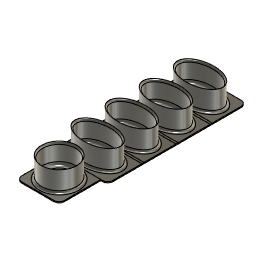
gluboost-organizer (Autodesk Fusion 360 design; units mm, degrees)
Autodesk Fusion 360 part; units mm, degrees
sketch "Sketch1" plane through (0, 0, 0) normal (0, 0, 1) x (1, 0, 0)
  ellipse E0 centre (0, 0) end of major axis (25.4, 0) minor radius 14.986
  line L0 (-25.4, 0) -> (25.4, 0)
  line L1 (0, -14.986) -> (0, 14.986)
  line L2 (33.6277, 21.621) -> (-33.6277, 21.621)
  line L3 (-33.6277, 21.621) -> (-33.6277, -21.621)
  line L4 (-33.6277, -21.621) -> (33.6277, -21.621)
  line L5 (33.6277, -21.621) -> (33.6277, 21.621)
  line L6 (33.6277, 21.621) -> (-33.6277, -21.621) construction
  line L7 (-33.6277, 21.621) -> (33.6277, -21.621) construction
  ellipse E1 centre (0, 0) end of major axis (27.1057, 0) minor radius 16.4243
  line L8 (-27.1057, 0) -> (27.1057, 0)
  line L9 (0, -16.4243) -> (0, 16.4243)
  line L10 (-25.4, -20.3918) -> (25.4, -71.1918) construction
  line L11 (25.4, -20.3918) -> (-25.4, -20.3918)
  circle A0 centre (0, -45.7918) radius 19.685
  line L12 (25.4, -71.1918) -> (25.4, -20.3918)
  line L13 (25.4, -20.3918) -> (-25.4, -71.1918) construction
  line L14 (-25.4, -20.3918) -> (-25.4, -71.1918)
  line L15 (-25.4, -71.1918) -> (25.4, -71.1918)
  circle A1 centre (0, -45.7918) radius 20.955
  point P0 (0, -45.7918)
  point P1 (0, -45.7918)
  dimension "d1" = 50.8
  dimension "d2" = 29.972
  dimension "d36" = 39.37
  dimension "d37" = 41.91
  dimension "d38" = 50.8
  constraint coincident E0.centre E1.centre
  constraint horizontal L0
  constraint coincident E0 L0.start
  constraint coincident E0 L0.end
  constraint coincident E0 L1.start
  constraint coincident E0 L1.end
  constraint horizontal L2
  constraint perpendicular L2 L3
  constraint parallel L2 L4
  constraint parallel L3 L5
  constraint coincident L6 E0.centre
  constraint coincident L7 E0.centre
  constraint parallel L0 L8
  constraint coincident E1 L8.start
  constraint coincident E1 L8.end
  constraint coincident E1 L9.start
  constraint coincident E1 L9.end
  constraint coincident P1 P0
  constraint concentric A0 A1
  constraint horizontal L11
  constraint perpendicular L11 L14
  constraint parallel L11 L15
  constraint parallel L12 L14
  constraint coincident P1 L13
  constraint coincident P1 L10
  measures "d1" distance of E0
  measures "d36" diameter of A0
  measures "d37" diameter of A1
  measures "d38" distance of L13.end L10.end
extrude "Extrude3" add sketch "Sketch1" along normal blind 1.27 contours E0 L0 L1 L8 L9 | E0 E1 L8 L9 | E0 L0 L1 L8 L9 | E0 E1 L8 L9 | E0 L0 L1 L8 L9 | E0 E1 L8 L9 | E0 E1 L8 L9 | E0 L0 L1 L8 L9 | L2 L3 L4 L5 L11 L12 L14 | L4 L11 L12 L14 makes body 1
extrude "Extrude4" add sketch "Sketch1" along normal blind 25.4 contours E0 E1 L8 L9 | E0 E1 L8 L9 | E0 E1 L8 L9 | E0 E1 L8 L9 bodies 1
fillet "Fillet4" radius 2.54 1 edges at (-25.4, 0, 25.4) on bodies 1
fillet "Fillet6" radius 3.81 1 edges at (-25.4, 0, 1.27) on bodies 1
pattern_linear "R-Pattern2" count 4 spacing 40.64 along (0, 1, 0) of bodies 1 makes body 2 at (11.2092, 47.847, 0) makes body 3 at (11.2092, 88.487, 0) makes body 4 at (11.2092, 129.127, 0)
extrude "Extrude6" add sketch "Sketch1" along normal blind 1.27 separate body contours L4 L12 L14 L15 | A0 | A1 makes body 5
fillet "Fillet9" radius 2.54 4 edges at (-27.1057, 0, 1.27) (-27.1057, 40.64, 1.27) (-27.1057, 81.28, 1.27) (-27.1057, 121.92, 1.27) on bodies 1 2 3 4
extrude "Extrude7" add sketch "Sketch1" along normal blind 25.4 contours A1 bodies 5
fillet "Fillet10" radius 3.175 1 edges at (-18.3529, -38.6734, 25.4) on bodies 5
fillet "Fillet11" radius 2.54 1 edges at (-19.5369, -38.2142, 1.27) on bodies 5
fillet "Fillet12" radius 6.35 6 edges at (-33.6277, -21.621, 0.635) (33.6277, -21.621, 0.635) (33.6277, 143.541, 0.635) (-33.6277, 143.541, 0.635) (-25.4, -71.1918, 0.635) (25.4, -71.1918, 0.635) on bodies 1 4 5
fillet "Fillet13" radius 3.81 1 edges at (-18.3529, -52.9102, 1.27) on bodies 5
pattern_linear "R-Pattern1" [suppressed]
extrude "Extrude5" [suppressed]
fillet "Fillet7" [suppressed]
extrude "Extrude1" [suppressed]
extrude "Extrude2" [suppressed]
fillet "Fillet1" [suppressed]
